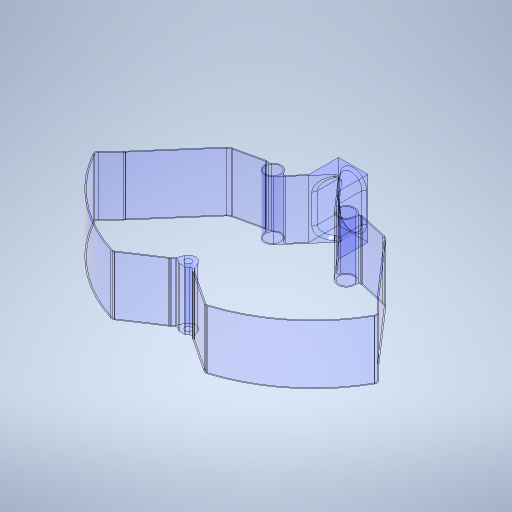
# Autodesk Inventor part: Top Plate
Saved by Autodesk Inventor 2023.2 (Build 272271000, 271)
## iProperties
Created: 2022-12-28
Part Number: Top Plate
Material: UHMW, White
Document SubType Name: Modeling
Designer: Nathan Cai
Mass: 7.48439 g
Surface Area: 194.835 cm^2
Volume: 7.96212 cm^3
Density: 0.94 g/cm^3
Appearance: Clear - Blue
Author: Nathan Cai
Autodesk Inventor part; units mm, degrees
ref_plane "YZ Plane" through (0, 0, 0) normal (1, 0, 0) x (0, 1, 0)
ref_plane "XZ Plane" through (0, 0, 0) normal (0, 1, 0) x (-1, 0, 0)
ref_plane "XY Plane" through (0, 0, 0) normal (0, 0, 1) x (1, 0, 0)
sketch "Sketch1" plane through (0, 0, 0) normal (0, 1, 0) x (-1, 0, 0)
  circle A0 centre (0, 0) radius 73.025
  line L0 (0, 0) -> (0, -73.025) construction
  line L1 (0, 0) -> (-12.6807, -71.9156)
  line L2 (0, 0) -> (12.6807, -71.9156)
  line L3 (0, 0) -> (52.5298, -50.7274)
  line L4 (0, 0) -> (32.0121, -65.6344)
  line L5 (0, 0) -> (72.3143, -10.1631)
  line L6 (0, 0) -> (64.4772, -34.2832)
  line L7 (0, 0) -> (64.4772, 34.2832)
  line L8 (0, 0) -> (72.3143, 10.1631)
  line L9 (0, 0) -> (32.0121, 65.6344)
  line L10 (0, 0) -> (52.5298, 50.7274)
  circle A1 centre (0, 0) radius 69.85
  line L11 (0, 0) -> (-12.6807, 71.9156)
  line L12 (0, 0) -> (12.6807, 71.9156)
  line L13 (0, 0) -> (-52.5298, 50.7274)
  line L14 (0, 0) -> (-32.0121, 65.6344)
  line L15 (0, 0) -> (-72.3143, 10.1631)
  line L16 (0, 0) -> (-64.4772, 34.2832)
  line L17 (0, 0) -> (-64.4772, -34.2832)
  line L18 (0, 0) -> (-72.3143, -10.1631)
  line L19 (0, 0) -> (-32.0121, -65.6344)
  line L20 (0, 0) -> (-52.5298, -50.7274)
  point P0 (30.6202, -62.7808)
  point P1 (50.2459, -48.5219)
  point P2 (52.5298, -50.7274)
  point P3 (64.4772, -34.2832)
  point P4 (61.6739, -32.7926)
  point P5 (69.1702, -9.7212)
  point P6 (72.3143, -10.1631)
  point P7 (72.3143, 10.1631)
  point P8 (69.1702, 9.7212)
  point P9 (61.6739, 32.7926)
  point P10 (52.5298, 50.7274)
  point P11 (50.2459, 48.5219)
  point P12 (30.6202, 62.7808)
  point P13 (-12.1293, -68.7888)
  point P14 (12.1293, -68.7888)
  point P15 (12.6807, -71.9156)
  point P16 (32.0121, -65.6344)
  point P17 (12.1293, 68.7888)
  point P18 (-12.1293, 68.7888)
  point P19 (-12.6807, 71.9156)
  point P20 (-64.4772, 34.2832)
  point P21 (-61.6739, 32.7926)
  point P22 (-69.1702, 9.7212)
  point P23 (-52.5298, -50.7274)
  point P24 (-50.2459, -48.5219)
  point P25 (-30.6202, -62.7808)
  dimension "d0" = 146.05
  dimension "d1" = 10
  dimension "d4" = 360
  dimension "d160" = 139.7
  constraints: 42 end point, 4 coincident, 2 centre point, 2 point on circle, 1 symmetric about line, 1 vertical, 49 other
  measures "d0" diameter of A0
  measures "d1" angle of L0 L1
  measures "d160" diameter of A1
extrude "Extrusion1" add sketch "Sketch1" along normal blind 3.175 contours A0 L5 A1 L8 | A0 L6 A1 L5 | L7 A1 L10 A0 | A1 L5 L8 | L8 L7 A1 | A0 L3 A1 L6 | A1 L6 L5 | L10 A1 L9 A0 | L7 L10 A1 | L2 A1 L1 | L4 A1 L2 | L6 A1 L3 | L3 A1 L4 | L12 A1 L9 | L9 A1 L10 | L14 A1 L11 | L11 A1 L12 | L16 A1 L13 | L13 A1 L14 | L18 A1 L15 | L15 A1 L16 | L20 A1 L17 | L17 A1 L18 | L1 A1 L19 | L19 A1 L20 | L9 A1 L12 A0 | A1 L2 A0 L1 | L1 A0 L19 A1 | A1 L4 A0 L2 | A1 L14 A0 L11 | L13 A0 L14 A1 | A1 L16 A0 L13 | A1 L18 A0 L15 | L17 A0 L18 A1 | A1 L20 A0 L17
sketch "Sketch4" plane through (0, 3.175, 0) normal (0, 1, 0) x (1, 0, 0)
  line L0 (0, 0) -> (0, 66.675) construction
  line L1 (-44.45, 30.1625) -> (44.45, 30.1625) construction
  line L2 (44.45, 30.1625) -> (44.45, 1.5875)
  line L3 (44.45, 1.5875) -> (-44.45, 1.5875) construction
  line L4 (-44.45, 1.5875) -> (-44.45, 30.1625)
  line L5 (-44.45, 30.1625) -> (44.45, 1.5875) construction
  line L6 (44.45, 30.1625) -> (-44.45, 1.5875) construction
  line L7 (-44.45, 15.875) -> (44.45, 15.875) construction
  line L8 (-60.325, 38.1) -> (-44.45, 38.1)
  line L9 (-44.45, 38.1) -> (-44.45, -6.35)
  line L10 (-44.45, -6.35) -> (-60.325, -6.35)
  line L11 (-60.325, -6.35) -> (-60.325, 38.1)
  line L12 (-60.325, 38.1) -> (-44.45, -6.35) construction
  line L13 (-44.45, 38.1) -> (-60.325, -6.35) construction
  line L14 (44.45, 1.5875) -> (44.45, 30.1625)
  line L15 (60.325, 38.1) -> (44.45, 38.1)
  line L16 (44.45, 38.1) -> (44.45, -6.35)
  line L17 (44.45, -6.35) -> (60.325, -6.35)
  line L18 (60.325, -6.35) -> (60.325, 38.1)
  line L19 (60.325, 38.1) -> (44.45, -6.35) construction
  line L20 (44.45, 38.1) -> (60.325, -6.35) construction
  line L21 (38.1, 15.875) -> (38.1, 31.75) construction
  circle A0 centre (38.1, 31.75) radius 1.7526
  circle A1 centre (38.1, 0) radius 1.7526
  circle A2 centre (-38.1, 31.75) radius 1.7526
  circle A3 centre (-38.1, 0) radius 1.7526
  line L22 (-60.325, 38.1) -> (-53.975, 38.1)
  line L23 (-53.975, 38.1) -> (-53.975, 31.75)
  line L24 (-53.975, 31.75) -> (-60.325, 31.75) construction
  line L25 (-60.325, 31.75) -> (-60.325, 38.1)
  line L26 (-53.975, 31.75) -> (-60.325, 28.0838)
  line L27 (-53.975, -6.35) -> (-53.975, 0)
  line L28 (-53.975, 0) -> (-60.325, 3.6662)
  line L29 (53.975, 38.1) -> (53.975, 31.75)
  line L30 (53.975, 31.75) -> (60.325, 28.0838)
  line L31 (53.975, -6.35) -> (53.975, 0)
  line L32 (53.975, 0) -> (60.325, 3.6662)
  line L33 (-38.1, 0) -> (38.1, 0) construction
  circle A4 centre (-15.875, -1.5875) radius 1.7526
  circle A5 centre (15.875, -1.5875) radius 1.7526
  line L34 (-21.3, 28.575) -> (-7.0125, 28.575)
  line L35 (-7.0125, 28.575) -> (-7.0125, 3.175)
  line L36 (-7.0125, 3.175) -> (-21.3, 3.175)
  line L37 (-21.3, 3.175) -> (-21.3, 28.575)
  line L38 (-21.3, 28.575) -> (-7.0125, 3.175) construction
  line L39 (-7.0125, 28.575) -> (-21.3, 3.175) construction
  line L40 (21.3, 28.575) -> (7.0125, 28.575)
  line L41 (7.0125, 28.575) -> (7.0125, 3.175)
  line L42 (7.0125, 3.175) -> (21.3, 3.175)
  line L43 (21.3, 3.175) -> (21.3, 28.575)
  line L44 (21.3, 28.575) -> (7.0125, 3.175) construction
  line L45 (7.0125, 28.575) -> (21.3, 3.175) construction
  circle A6 centre (25.4944, -54.673) radius 3.175
  line L46 (25.4944, -54.673) -> (31.5337, -52.7108) construction
  circle A7 centre (31.5337, -52.7108) radius 1.5875
  line L47 (25.4944, -54.673) -> (25.4944, -51.498) construction
  circle A8 centre (30.2134, -58.922) radius 1.5875
  circle A9 centre (24.1742, -60.8843) radius 1.5875
  circle A10 centre (19.4552, -56.6353) radius 1.5875
  circle A11 centre (20.7755, -50.424) radius 1.5875
  circle A12 centre (26.8147, -48.4618) radius 1.5875
  circle A13 centre (-25.4944, -54.673) radius 3.175
  line L48 (-25.4944, -54.673) -> (-31.5337, -52.7108) construction
  circle A14 centre (-31.5337, -52.7108) radius 1.5875
  line L49 (-25.4944, -54.673) -> (-25.4944, -51.498) construction
  circle A15 centre (-30.2134, -58.922) radius 1.5875
  circle A16 centre (-24.1742, -60.8843) radius 1.5875
  circle A17 centre (-19.4552, -56.6353) radius 1.5875
  circle A18 centre (-20.7755, -50.424) radius 1.5875
  circle A19 centre (-26.8147, -48.4618) radius 1.5875
  circle A20 centre (0, 0) radius 60.325 construction
  line L50 (0, 0) -> (25.4944, -54.673) construction
  circle A21 centre (25.4944, -54.673) radius 9.525 construction
  circle A22 centre (31.75, 38.1) radius 3.175
  circle A23 centre (-31.75, 38.1) radius 3.175
  point P0 (0, 15.875)
  point P1 (-52.3875, 15.875)
  point P2 (52.3875, 15.875)
  point P3 (0, 15.875)
  point P4 (-60.325, 3.6662)
  point P5 (-53.975, -6.35)
  point P6 (-53.975, 38.1)
  point P7 (53.975, -6.35)
  point P8 (60.325, 3.6662)
  point P9 (53.975, 38.1)
  point P10 (-14.1563, 15.875)
  point P11 (14.1563, 15.875)
  dimension "d108" = 6.35
  dimension "d173" = 120.65
  dimension "d30" = 88.9
  dimension "d31" = 28.575
  dimension "d34" = 15.875
  dimension "d35" = 44.45
  dimension "d52" = 6.35
  dimension "d53" = 15.875
  dimension "d54" = 3.5052
  dimension "d63" = 15.875
  dimension "d64" = 6.35
  dimension "d65" = 6.35
  dimension "d66" = 30
  dimension "d78" = 3.5052
  dimension "d79" = 15.875
  dimension "d80" = 17.4625
  dimension "d104" = 14.2875
  dimension "d105" = 25.4
  dimension "d107" = 23.15
  dimension "d111" = 6.35
  dimension "d112" = 3.175
  dimension "d113" = 72
  dimension "d116" = 360
  dimension "d174" = 25
  dimension "d175" = 19.05
  dimension "d176" = 6.35
  dimension "d177" = 22.225
  dimension "d178" = 31.75
  constraints: 102 end point, 33 symmetric about line, 21 centre point, 11 midpoint, 8 parallel, 5 coincident, 5 horizontal, 5 point on line, 4 perpendicular, 4 vertical, 2 vertical alignment, 31 other
  measures "d30" distance of L2.end L3.end
  measures "d31" distance between parallel lines of L3 L1
  measures "d34" distance of L9.end L10.end
  measures "d35" distance of L8.end L9.end
  measures "d52" distance between parallel lines of L16 L21
  measures "d53" distance from line of L7 L21.end
  measures "d54" diameter of A0
  measures "d63" distance of point (0, 15.875) L0.start
  measures "d64" distance of L23.end L24.end
  measures "d65" distance of L22.end L23.end
  measures "d66" angle of L24 L26
  measures "d78" diameter of A4
  measures "d79" distance from line of L0 A4.centre
  measures "d80" distance from line of L7 A4.centre
  measures "d104" distance of L35.end L36.end
  measures "d105" distance of L34.end L35.end
  measures "d107" distance between parallel lines of L4 L37
  measures "d111" distance of L46.start L46.end
  measures "d112" diameter of A7
  measures "d113" angle of L47 L46
  measures "d174" angle of L0 L50
  measures "d175" diameter of A21
  measures "d176" diameter of A22
  measures "d177" vertical distance of point (0, 15.875) A22.centre
  measures "d178" distance from line of L0 A22.centre
extrude "Extrusion2" cut sketch "Sketch4" against normal through all
fillet "Fillet2" radius 4.7625 16 edges at (-44.45, 1.5875, -38.1) (-44.45, 1.5875, 6.35) (44.45, 1.5875, 6.35) (44.45, 1.5875, -38.1) (-21.3, 1.5875, -28.575) (-7.0125, 1.5875, -28.575) (-7.0125, 1.5875, -3.175) (-21.3, 1.5875, -3.175) (7.0125, 1.5875, -28.575) (21.3, 1.5875, -28.575) (21.3, 1.5875, -3.175) (7.0125, 1.5875, -3.175) (60.325, 1.5875, -38.1) (60.325, 1.5875, 6.35) (-60.325, 1.5875, -38.1) (-60.325, 1.5875, 6.35)
sketch "Sketch5" plane through (0, 3.175, 0) normal (0, 1, 0) x (1, 0, 0)
  line L0 (0, 0) -> (0, 66.675) construction
  circle A0 centre (0, 50.8) radius 22.225
  arc A1 (32.0121, 65.6344) -> (-32.0121, 65.6344) centre (0, 0) ccw projected
  circle A2 centre (0, 50.8) radius 17.4625 construction
  circle A3 centre (-24.6063, 60.325) radius 1.7526
  circle A4 centre (-24.6063, 60.325) radius 3.175 construction
  circle A5 centre (-22.225, 34.925) radius 3.175 construction
  circle A6 centre (-22.225, 34.925) radius 1.7526
  circle A7 centre (24.6063, 60.325) radius 1.7526
  circle A8 centre (24.6063, 60.325) radius 3.175 construction
  circle A9 centre (22.225, 34.925) radius 3.175 construction
  circle A10 centre (22.225, 34.925) radius 1.7526
  arc A11 (32.0121, 65.6344) -> (-32.0121, 65.6344) centre (0, 0) ccw projected
  line L1 (-19.05, 70.4964) -> (-21.8767, 54.7195)
  line L2 (19.05, 70.4964) -> (21.8767, 54.7195)
  circle A12 centre (0, 28.575) radius 4.7625
  line L3 (0, 33.3375) -> (0, 23.8125) construction
  line L4 (-4.7625, 33.3375) -> (-4.7625, 23.8125)
  line L5 (4.7625, 23.8125) -> (4.7625, 33.3375)
  arc A13 (4.7625, 33.3375) -> (-4.7625, 33.3375) centre (0, 33.3375) ccw
  arc A14 (-4.7625, 23.8125) -> (4.7625, 23.8125) centre (0, 23.8125) ccw
  point P0 (-30.5456, -66.3296)
  point P1 (12.6807, -71.9156)
  point P2 (64.4772, -34.2832)
  point P3 (-72.5223, -8.5536)
  point P4 (-19.05, 70.4964)
  point P5 (0, 73.025)
  point P6 (21.8767, 54.7195)
  point P7 (19.05, 70.4964)
  point P8 (-4.7351, 29.0853)
  point P9 (4.7351, 29.0853)
  point P10 (0, 19.05)
  point P11 (4.7625, 28.575)
  point P12 (-4.7625, 28.575)
  dimension "d39" = 34.925
  dimension "d40" = 44.45
  dimension "d41" = 3.5052
  dimension "d42" = 6.35
  dimension "d43" = 9.525
  dimension "d44" = 24.6062
  dimension "d45" = 6.35
  dimension "d46" = 3.5052
  dimension "d47" = 15.875
  dimension "d48" = 22.225
  dimension "d74" = 19.05
  dimension "d102" = 9.525
  dimension "d103" = 9.525
  constraints: 14 end point, 13 centre point, 8 point on circle, 7 tangent, 6 symmetric about line, 5 coincident, 3 point on line, 1 midpoint, 1 parallel, 1 vertical, 4 other
  measures "d39" diameter of A2
  measures "d40" diameter of A0
  measures "d41" diameter of A3
  measures "d42" diameter of A4
  measures "d43" vertical distance of A0.centre A3.centre
  measures "d44" horizontal distance of A0.centre A3.centre
  measures "d45" diameter of A5
  measures "d46" diameter of A6
  measures "d47" vertical distance of A0.centre A6.centre
  measures "d48" horizontal distance of A0.centre A6.centre
  measures "d74" distance from line of L0 L1.start
  measures "d102" diameter of A12
  measures "d103" distance of point (0, 19.05) A12.centre
extrude "Extrusion3" cut sketch "Sketch5" against normal blind 25.4 contours A0 L5 A13 L4 | A0 A1 L2 | A0 A12 L4 A13 L5 | A0 L1 A1 | A12 A0 | A0 A12 | L5 A14 L4 A12 | A3 | A6 | A7 | A10
sketch "Sketch6" plane through (0, 0, 0) normal (0, -1, 0) x (1, 0, 0)
  point P0 (11.8537, 67.2254)
  point P1 (-11.8537, 67.2254)
hole "Hole3" at (11.8537, 0, 67.2254) at (-11.8537, 0, 67.2254) direction (0, 1, 0) diameter 3.5052 end through all
sketch "Sketch7" plane through (0, 3.175, 0) normal (0, 1, 0) x (1, 0, 0)
  arc A0 (12.158, -68.9514) -> (11.3889, -68.9153) centre (11.8537, -67.2254) ccw projected
  circle A1 centre (11.8537, -67.2254) radius 3.302
  arc A2 (-11.3889, -68.9153) -> (-12.158, -68.9514) centre (-11.8537, -67.2254) ccw projected
  circle A3 centre (-11.8537, -67.2254) radius 3.302
  circle A4 centre (11.8537, -67.2254) radius 1.7526
  circle A5 centre (-11.8537, -67.2254) radius 1.7526
  point P0 (0, 0)
  point P1 (12.158, -68.9514)
  point P2 (11.3889, -68.9153)
  dimension "d67" = 6.604
  dimension "d68" = 6.604
  constraints: 4 coincident, 3 centre point, 1 concentric, 3 other
  measures "d67" diameter of A1
  measures "d68" diameter of A3
extrude "Extrusion4" add sketch "Sketch7" against normal up to surface (3.175 mm away)
fillet "Fillet4" radius 1.5875 24 edges at (-12.6807, 1.5875, 71.9156) (-12.427, 1.5875, 70.4773) (-9.235, 1.5875, 69.2368) (12.6807, 1.5875, 71.9156) (12.427, 1.5875, 70.4773) (9.235, 1.5875, 69.2368) (69.1702, 1.5875, 9.7212) (72.3143, 1.5875, 10.1631) (64.4772, 1.5875, 34.2832) (61.6739, 1.5875, 32.7926) (30.6202, 1.5875, -62.7808) (32.0121, 1.5875, -65.6344) (52.5298, 1.5875, -50.7274) (50.2459, 1.5875, -48.5219) (-32.0121, 1.5875, -65.6344) (-30.6202, 1.5875, -62.7808) (-52.5298, 1.5875, -50.7274) (-50.2459, 1.5875, -48.5219) (-72.3143, 1.5875, 10.1631) (-69.1702, 1.5875, 9.7212) (-61.6739, 1.5875, 32.7926) (-64.4772, 1.5875, 34.2832) (-4.7351, 1.5875, -29.0853) (4.7351, 1.5875, -29.0853)
fillet "Fillet5" radius 3.175 2 edges at (19.05, 1.5875, -70.4964) (-19.05, 1.5875, -70.4964)
thicken "Thicken1" operation cut thickness 0.25 both sides no extend neighbours no toward (-0.8477101, 0, -0.5304598) faces at (61.904, 2.1167, 38.7368) (63.0601, 1.0583, 33.5296) (63.8199, 1.0583, 34.4266) (13.1942, 1.0583, 71.6582) (62.9587, 1.0583, 33.4709) (12.2225, 1.0583, 70.9396) (66.7871, 2.1167, 20.4576) (9.8443, 2.1167, 69.8457) (70.7248, 1.0583, 9.9397) (69.8129, 1.0583, 10.0825) (8.7126, 2.1167, 69.3268) (70.965, 1.0583, 9.9551) (6.579, 2.1167, 69.5395) (62.1056, 2.1167, -38.4128) (-8.7126, 2.1167, 69.3268) (51.3752, 1.0583, -49.6125) (52.5834, 1.0583, -50.0545) (-9.8443, 1.0583, 69.8457) (50.9955, 1.0583, -49.3411) (-11.7264, 1.0583, 70.5997) (40.0946, 2.1167, -57.1965) (-12.915, 1.0583, 71.5521) (31.3084, 1.0583, -64.1918) (31.1624, 1.0583, -63.2804) (-45.5793, 2.1167, 57.0541) (31.3571, 1.0583, -64.302) (-63.06, 1.0583, 33.5296) (-63.6672, 1.0583, 34.1) (24.8679, 2.1167, -68.6603) (-62.2411, 1.0583, 31.857) (-63.4147, 2.1167, 29.2848) (-70.7249, 1.0583, 9.9397) (-70.2583, 1.0583, 9.9434) (-72.3414, 1.0583, 9.1242) (-72.823, 2.1167, -5.4282) (-51.3752, 1.0583, -49.6124) (-51.8764, 1.0583, -49.9396) (-49.8575, 1.0583, -49.222) (-42.0072, 2.1167, -55.807) (-31.3084, 1.0583, -64.1918) (-31.8083, 1.0583, -62.207) (-31.1844, 1.0583, -65.7948) (-29.847, 2.1167, -66.6469) (19.9211, 2.1167, -65.8489) (21.2411, 2.1167, -58.2668) (13.984, 1.0583, -33.5258) (5.2423, 1.0583, -28.987) (4.7625, 2.1167, -25.1583) (-4.3814, 1.0583, -21.9458) (-4.7625, 1.0583, -26.5041) (-5.421, 1.0583, -29.1371) (-19.7168, 1.0583, -40.5434) (-20.6056, 2.1167, -61.8142) (-19.9361, 2.1167, -65.6043)
sketch "Sketch11" plane through (0, 3.175, 0) normal (0, 1, 0) x (1, 0, 0)
  line L0 (-26.9875, -14.2875) -> (-7.9375, -14.2875) construction
  line L1 (-26.9875, -16.6688) -> (-7.9375, -16.6688)
  line L2 (-7.9375, -11.9062) -> (-26.9875, -11.9063)
  arc A0 (-26.9875, -11.9063) -> (-26.9875, -16.6688) centre (-26.9875, -14.2875) ccw
  arc A1 (-7.9375, -16.6688) -> (-7.9375, -11.9062) centre (-7.9375, -14.2875) ccw
  line L3 (-17.4625, -14.2875) -> (-17.4625, -39.6875) construction
  line L4 (-23.8125, -26.9875) -> (-11.1125, -26.9875) construction
  line L5 (-23.8125, -29.3688) -> (-11.1125, -29.3687)
  line L6 (-11.1125, -24.6062) -> (-23.8125, -24.6062)
  arc A2 (-23.8125, -24.6062) -> (-23.8125, -29.3688) centre (-23.8125, -26.9875) ccw
  arc A3 (-11.1125, -29.3687) -> (-11.1125, -24.6062) centre (-11.1125, -26.9875) ccw
  line L7 (-30.1625, -39.6875) -> (-4.7625, -39.6875) construction
  line L8 (-30.1625, -42.0688) -> (-4.7625, -42.0688)
  line L9 (-4.7625, -37.3062) -> (-30.1625, -37.3063)
  arc A4 (-30.1625, -37.3063) -> (-30.1625, -42.0688) centre (-30.1625, -39.6875) ccw
  arc A5 (-4.7625, -42.0688) -> (-4.7625, -37.3062) centre (-4.7625, -39.6875) ccw
  circle A6 centre (-11.1125, -33.3375) radius 2.3813
  line L10 (-17.4625, -39.6875) -> (-17.4625, -14.2875) construction
  line L11 (-15.0813, -39.6875) -> (-15.0812, -14.2875)
  line L12 (-19.8438, -14.2875) -> (-19.8438, -39.6875)
  arc A7 (-19.8438, -39.6875) -> (-15.0813, -39.6875) centre (-17.4625, -39.6875) ccw construction
  arc A8 (-15.0812, -14.2875) -> (-19.8438, -14.2875) centre (-17.4625, -14.2875) ccw construction
  line L13 (20.6375, -14.2875) -> (20.6375, -39.6875) construction
  circle A9 centre (14.2875, -14.2875) radius 2.3813 construction
  line L14 (15.875, -20.6375) -> (15.875, -26.9875) construction
  line L15 (13.4938, -20.6375) -> (13.4938, -26.9875)
  line L16 (18.2563, -26.9875) -> (18.2563, -20.6375)
  arc A10 (18.2563, -20.6375) -> (13.4938, -20.6375) centre (15.875, -20.6375) ccw
  arc A11 (13.4938, -26.9875) -> (18.2563, -26.9875) centre (15.875, -26.9875) ccw
  line L17 (15.875, -20.6375) -> (25.4, -20.6375) construction
  line L18 (15.875, -23.0187) -> (25.4, -23.0187)
  line L19 (25.4, -18.2562) -> (15.875, -18.2562)
  arc A12 (15.875, -18.2562) -> (15.875, -23.0187) centre (15.875, -20.6375) ccw
  arc A13 (25.4, -23.0187) -> (25.4, -18.2562) centre (25.4, -20.6375) ccw
  line L20 (15.875, -26.9875) -> (25.4, -26.9875) construction
  line L21 (15.875, -24.6062) -> (25.4, -24.6062)
  line L22 (25.4, -29.3687) -> (15.875, -29.3687)
  arc A14 (15.875, -24.6062) -> (15.875, -29.3687) centre (15.875, -26.9875) ccw
  arc A15 (25.4, -29.3687) -> (25.4, -24.6062) centre (25.4, -26.9875) ccw
  circle A16 centre (26.9875, -14.2875) radius 2.3813 construction
  line L23 (26.9875, -14.2875) -> (30.1625, -8.7882) construction
  line L24 (29.0497, -15.4781) -> (32.2247, -9.9789)
  line L25 (28.1003, -7.5976) -> (24.9253, -13.0969)
  arc A17 (24.9253, -13.0969) -> (29.0497, -15.4781) centre (26.9875, -14.2875) ccw
  arc A18 (32.2247, -9.9789) -> (28.1003, -7.5976) centre (30.1625, -8.7882) ccw
  line L26 (26.9875, -14.2875) -> (33.3375, -14.2875) construction
  line L27 (14.2875, -14.2875) -> (11.1125, -8.7882) construction
  line L28 (16.3497, -13.0969) -> (13.1747, -7.5976)
  line L29 (9.0503, -9.9789) -> (12.2253, -15.4781)
  arc A19 (12.2253, -15.4781) -> (16.3497, -13.0969) centre (14.2875, -14.2875) ccw
  arc A20 (13.1747, -7.5976) -> (9.0503, -9.9789) centre (11.1125, -8.7882) ccw
  line L30 (14.2875, -14.2875) -> (20.6375, -14.2875) construction
  line L31 (11.1125, -33.3375) -> (11.1125, -39.6875) construction
  line L32 (8.7313, -33.3375) -> (8.7313, -39.6875)
  line L33 (13.4938, -39.6875) -> (13.4938, -33.3375)
  arc A21 (13.4938, -33.3375) -> (8.7313, -33.3375) centre (11.1125, -33.3375) ccw
  arc A22 (8.7313, -39.6875) -> (13.4938, -39.6875) centre (11.1125, -39.6875) ccw
  line L34 (17.4625, -33.3375) -> (17.4625, -39.6875) construction
  line L35 (15.0813, -33.3375) -> (15.0813, -39.6875)
  line L36 (19.8438, -39.6875) -> (19.8438, -33.3375)
  arc A23 (19.8438, -33.3375) -> (15.0813, -33.3375) centre (17.4625, -33.3375) ccw
  arc A24 (15.0813, -39.6875) -> (19.8438, -39.6875) centre (17.4625, -39.6875) ccw
  line L37 (17.4625, -39.6875) -> (30.1625, -39.6875) construction
  line L38 (17.4625, -37.3062) -> (30.1625, -37.3062)
  line L39 (30.1625, -42.0688) -> (17.4625, -42.0688)
  arc A25 (17.4625, -37.3062) -> (17.4625, -42.0688) centre (17.4625, -39.6875) ccw
  arc A26 (30.1625, -42.0688) -> (30.1625, -37.3062) centre (30.1625, -39.6875) ccw
  circle A27 centre (23.8125, -33.3375) radius 2.3813
  circle A28 centre (30.1625, -33.3375) radius 2.3813
  line L40 (17.4625, -33.3375) -> (30.1625, -33.3375) construction
  line L41 (30.1625, -33.3375) -> (30.1625, -39.6875) construction
  arc A29 (53.6121, -36.9069) -> (36.9069, -53.6121) centre (52.759, -52.759) ccw construction
  arc A30 (53.7828, -33.7365) -> (33.7365, -53.7828) centre (52.759, -52.759) ccw
  arc A31 (53.4415, -40.0774) -> (40.0774, -53.4415) centre (52.759, -52.759) ccw
  arc A32 (53.4415, -40.0774) -> (53.7828, -33.7365) centre (53.6121, -36.9069) ccw
  arc A33 (33.7365, -53.7828) -> (40.0774, -53.4415) centre (36.9069, -53.6121) ccw
  circle A34 centre (0, 0) radius 65.0875 construction
  line L42 (0, 0) -> (41.5337, -41.5337) construction
  circle A35 centre (0, -64.525) radius 3 projected
  line L43 (0, 0) -> (0, -64.525) construction
  circle A36 centre (52.759, -52.759) radius 9.525
  arc A37 (-36.9069, -53.6121) -> (-53.6121, -36.9069) centre (-52.759, -52.759) ccw construction
  arc A38 (-33.7365, -53.7828) -> (-53.7828, -33.7365) centre (-52.759, -52.759) ccw
  arc A39 (-40.0774, -53.4415) -> (-53.4415, -40.0774) centre (-52.759, -52.759) ccw
  arc A40 (-53.7828, -33.7365) -> (-53.4415, -40.0774) centre (-53.6121, -36.9069) ccw
  arc A41 (-40.0774, -53.4415) -> (-33.7365, -53.7828) centre (-36.9069, -53.6121) ccw
  circle A42 centre (-52.759, -52.759) radius 9.525
  point P0 (-17.4625, -26.9875)
  point P1 (15.875, -23.8125)
  point P2 (20.6375, -20.6375)
  point P3 (20.6375, -26.9875)
  point P4 (20.6375, -26.9875)
  point P5 (28.575, -11.5379)
  point P6 (12.7, -11.5379)
  point P7 (11.1125, -36.5125)
  point P8 (17.4625, -36.5125)
  point P9 (23.8125, -39.6875)
  point P10 (-19.8438, -29.3688)
  point P11 (-19.8438, -37.3062)
  point P12 (-15.0813, -37.3062)
  point P13 (-15.0813, -29.3687)
  point P14 (-15.0812, -24.6062)
  point P15 (-15.0812, -16.6688)
  point P16 (-19.8438, -16.6688)
  point P17 (-19.8438, -24.6062)
  point P18 (15.875, -18.2562)
  point P19 (18.2563, -24.6062)
  point P20 (18.2563, -23.0187)
  point P21 (19.8438, -37.3062)
  dimension "d118" = 9.525
  dimension "d119" = 4.7625
  dimension "d120" = 25.4
  dimension "d121" = 2.3813
  dimension "d122" = 6.35
  dimension "d123" = 2.3813
  dimension "d124" = 12.7
  dimension "d125" = 4.7625
  dimension "d126" = 6.35
  dimension "d127" = 6.35
  dimension "d128" = 26.9875
  dimension "d129" = 17.4625
  dimension "d130" = 2.3813
  dimension "d131" = 20.6375
  dimension "d132" = 4.7625
  dimension "d133" = 3.175
  dimension "d134" = 4.7625
  dimension "d135" = 4.7625
  dimension "d136" = 2.3813
  dimension "d137" = 26.9875
  dimension "d138" = 6.35
  dimension "d139" = 6.35
  dimension "d140" = 6.35
  dimension "d141" = 60
  dimension "d142" = 6.35
  dimension "d143" = 120
  dimension "d144" = 2.3813
  dimension "d145" = 2.3813
  dimension "d146" = 3.175
  dimension "d147" = 25.4
  dimension "d148" = 6.35
  dimension "d149" = 6.35
  dimension "d150" = 4.7625
  dimension "d151" = 4.7625
  dimension "d152" = 6.35
  dimension "d155" = 6.35
  dimension "d156" = 130.175
  dimension "d157" = 15.875
  dimension "d158" = 45
  dimension "d159" = 19.05
  constraints: 112 end point, 74 point on circle, 53 tangent, 42 centre point, 17 equal length, 16 midpoint, 8 symmetric about line, 6 horizontal, 6 point on line, 5 vertical, 4 coincident, 3 perpendicular, 2 concentric, 6 other
  measures "d118" distance of L3.start L0.end
  measures "d119" diameter of A1
  measures "d120" distance of L3.start L3.end
  measures "d121" radius of A3
  measures "d122" distance of L4.end point (-17.463, -26.988)
  measures "d123" radius of A5
  measures "d124" distance of L7.end L3.end
  measures "d125" diameter of A6
  measures "d126" distance from line of L3 A6.centre
  measures "d127" distance from line of L4 A6.centre
  measures "d128" vertical distance of point (0, 0) point (-17.463, -26.988)
  measures "d129" horizontal distance of point (0, 0) point (-17.463, -26.988)
  measures "d130" radius of A8
  measures "d131" horizontal distance of point (20.638, -26.988) point (0, 0)
  measures "d132" diameter of A9
  measures "d133" distance of point (15.875, -23.812) L14.end
  measures "d134" diameter of A16
  measures "d135" distance between parallel lines of L13 L14
  measures "d136" radius of A13
  measures "d137" vertical distance of point (0, 0) point (20.638, -26.988)
  measures "d138" distance from line of L13 L27.start
  measures "d139" distance from line of L13 L23.start
  measures "d140" distance of L23.start L23.end
  measures "d141" angle of L26 L23
  measures "d142" distance of L27.start L27.end
  measures "d143" angle of L30 L27
  measures "d144" radius of A26
  measures "d145" radius of A21
  measures "d146" distance between parallel lines of L34 L13
  measures "d147" distance of L13.start L13.end
  measures "d148" distance of L34.end L34.start
  measures "d149" distance of L37.end point (23.813, -39.688)
  measures "d150" diameter of A27
  measures "d151" diameter of A28
  measures "d152" distance between parallel lines of L34 L31
  measures "d155" diameter of A33
  measures "d156" diameter of A34
  measures "d157" radius of A29
  measures "d158" angle of L43 L42
  measures "d159" diameter of A36
extrude "Extrusion5" [suppressed]
sketch "Sketch13" plane through (0, 3.175, 0) normal (0, 1, 0) x (1, 0, 0)
  circle A0 centre (0, -65.0875) radius 7.9375 construction
  line L0 (0, 0) -> (0, -73.025) construction
  circle A1 centre (0, -53.975) radius 3.175
  circle A2 centre (0, -53.975) radius 1.7526
  circle A3 centre (0, 0) radius 73.025 construction
  dimension "d168" = 15.875
  dimension "d212" = 146.05
  dimension "d170" = 6.35
  dimension "d210" = 3.5052
  constraints: 2 centre point, 2 coincident, 2 end point, 2 point on line, 2 vertical alignment, 1 vertical, 4 other
  measures "d170" diameter of A1
  measures "d210" diameter of A2
extrude "Extrusion6" cut sketch "Sketch13" against normal through all contours A2
sketch "Sketch14" plane through (0, 3.175, 0) normal (0, 1, 0) x (1, 0, 0)
  arc A0 (-8.4203, -69.0888) -> (-9.8493, -69.5271) centre (-8.6426, -70.9128) ccw projected
  arc A1 (-8.4203, -69.0888) -> (8.4203, -69.0888) centre (0, 0) ccw projected
  arc A2 (9.8493, -69.5271) -> (8.4203, -69.0888) centre (8.6426, -70.9128) ccw projected
  arc A3 (9.8493, -69.5271) -> (11.3791, -70.2403) centre (11.8537, -67.2254) ccw projected
  arc A4 (12.5534, -70.9399) -> (11.3791, -70.2403) centre (11.0933, -72.0555) ccw projected
  arc A5 (12.5534, -70.9399) -> (13.8711, -71.4408) centre (13.6162, -70.1278) ccw projected
  arc A6 (13.8711, -71.4408) -> (63.4814, -35.5853) centre (0, 0) ccw projected
  arc A7 (63.4814, -35.5853) -> (62.9426, -33.7503) centre (62.3147, -34.9313) ccw projected
  arc A8 (62.1641, -31.3015) -> (62.9426, -33.7503) centre (63.8053, -32.1279) ccw projected
  arc A9 (62.1641, -31.3015) -> (68.6904, -11.2157) centre (0, 0) ccw projected
  arc A10 (70.7596, -9.6922) -> (68.6904, -11.2157) centre (70.5039, -11.5118) ccw projected
  arc A11 (70.7596, -9.6922) -> (72.274, -8.5243) centre (70.9457, -8.3677) ccw projected
  arc A12 (72.274, -8.5243) -> (53.4604, 49.3779) centre (0, 0) ccw projected
  arc A13 (53.4604, 49.3779) -> (51.5488, 49.4326) centre (52.4779, 48.4705) ccw projected
  arc A14 (48.9793, 49.4489) -> (51.5488, 49.4326) centre (50.2724, 50.7544) ccw projected
  arc A15 (48.9793, 49.4489) -> (31.8932, 61.8626) centre (0, 0) ccw projected
  arc A16 (31.0837, 64.3013) -> (31.8932, 61.8626) centre (32.7352, 63.4958) ccw projected
  arc A17 (31.0837, 64.3013) -> (30.441, 66.1025) centre (29.8816, 64.8877) ccw projected
  arc A18 (30.441, 66.1025) -> (24.0624, 68.6819) centre (0, 0) ccw projected
  arc A19 (24.0624, 68.6819) -> (20.2161, 65.4056) centre (23.0952, 65.9214) ccw projected
  line L0 (20.2161, 65.4056) -> (22.1227, 54.7636) projected
  arc A20 (5.9933, 29.1388) -> (22.1227, 54.7636) centre (0, 50.8) ccw projected
  arc A21 (5.9933, 29.1388) -> (5.0125, 27.8498) centre (6.35, 27.8498) ccw projected
  line L1 (5.0125, 27.8498) -> (5.0125, 23.8125) projected
  arc A22 (-5.0125, 23.8125) -> (5.0125, 23.8125) centre (0, 23.8125) ccw projected
  line L2 (-5.0125, 23.8125) -> (-5.0125, 27.8498) projected
  arc A23 (-5.0125, 27.8498) -> (-5.9933, 29.1388) centre (-6.35, 27.8498) ccw projected
  arc A24 (-22.1227, 54.7636) -> (-5.9933, 29.1388) centre (0, 50.8) ccw projected
  line L3 (-22.1227, 54.7636) -> (-20.2161, 65.4056) projected
  arc A25 (-20.2161, 65.4056) -> (-24.0624, 68.6819) centre (-23.0952, 65.9214) ccw projected
  arc A26 (-24.0624, 68.6819) -> (-30.441, 66.1025) centre (0, 0) ccw projected
  arc A27 (-30.441, 66.1025) -> (-31.0837, 64.3013) centre (-29.8816, 64.8877) ccw projected
  arc A28 (-31.8932, 61.8626) -> (-31.0837, 64.3013) centre (-32.7352, 63.4958) ccw projected
  arc A29 (-31.8932, 61.8626) -> (-48.9793, 49.4489) centre (0, 0) ccw projected
  arc A30 (-51.5488, 49.4326) -> (-48.9793, 49.4489) centre (-50.2724, 50.7544) ccw projected
  arc A31 (-51.5488, 49.4326) -> (-53.4604, 49.3779) centre (-52.4779, 48.4705) ccw projected
  arc A32 (-53.4604, 49.3779) -> (-72.274, -8.5243) centre (0, 0) ccw projected
  arc A33 (-72.274, -8.5243) -> (-70.7596, -9.6922) centre (-70.9457, -8.3677) ccw projected
  arc A34 (-68.6904, -11.2157) -> (-70.7596, -9.6922) centre (-70.5039, -11.5118) ccw projected
  arc A35 (-68.6904, -11.2157) -> (-62.1641, -31.3015) centre (0, 0) ccw projected
  arc A36 (-62.9426, -33.7503) -> (-62.1641, -31.3015) centre (-63.8053, -32.1279) ccw projected
  arc A37 (-62.9426, -33.7503) -> (-63.4814, -35.5853) centre (-62.3147, -34.9313) ccw projected
  arc A38 (-63.4814, -35.5853) -> (-13.8711, -71.4408) centre (0, 0) ccw projected
  arc A39 (-13.8711, -71.4408) -> (-12.5534, -70.9399) centre (-13.6162, -70.1278) ccw projected
  arc A40 (-11.3791, -70.2403) -> (-12.5534, -70.9399) centre (-11.0933, -72.0555) ccw projected
  arc A41 (-11.3791, -70.2403) -> (-9.8493, -69.5271) centre (-11.8537, -67.2254) ccw projected
  circle A42 centre (11.8537, -67.2254) radius 1.7526 projected
  circle A43 centre (-11.8537, -67.2254) radius 1.7526 projected
  circle A44 centre (31.75, 38.1) radius 3.175 projected
  circle A45 centre (25.4944, -54.673) radius 3.175 projected
  circle A46 centre (24.1742, -60.8843) radius 1.5875 projected
  circle A47 centre (-31.5337, -52.7108) radius 1.5875 projected
  line L4 (-7.0125, 23.8125) -> (-7.0125, 7.9375) projected
  arc A48 (-11.775, 3.175) -> (-7.0125, 7.9375) centre (-11.775, 7.9375) ccw projected
  line L5 (-11.775, 3.175) -> (-16.5375, 3.175) projected
  arc A49 (-21.3, 7.9375) -> (-16.5375, 3.175) centre (-16.5375, 7.9375) ccw projected
  line L6 (-21.3, 7.9375) -> (-21.3, 23.8125) projected
  arc A50 (-16.5375, 28.575) -> (-21.3, 23.8125) centre (-16.5375, 23.8125) ccw projected
  line L7 (-16.5375, 28.575) -> (-11.775, 28.575) projected
  arc A51 (-7.0125, 23.8125) -> (-11.775, 28.575) centre (-11.775, 23.8125) ccw projected
  line L8 (49.2125, 38.1) -> (55.5625, 38.1) projected
  arc A52 (60.325, 33.3375) -> (55.5625, 38.1) centre (55.5625, 33.3375) ccw projected
  line L9 (60.325, 33.3375) -> (60.325, -1.5875) projected
  arc A53 (55.5625, -6.35) -> (60.325, -1.5875) centre (55.5625, -1.5875) ccw projected
  line L10 (55.5625, -6.35) -> (49.2125, -6.35) projected
  arc A54 (44.45, -1.5875) -> (49.2125, -6.35) centre (49.2125, -1.5875) ccw projected
  line L11 (44.45, -1.5875) -> (44.45, 33.3375) projected
  arc A55 (49.2125, 38.1) -> (44.45, 33.3375) centre (49.2125, 33.3375) ccw projected
  circle A56 centre (38.1, 0) radius 1.7526 projected
  circle A57 centre (-38.1, 0) radius 1.7526 projected
  circle A58 centre (15.875, -1.5875) radius 1.7526 projected
  circle A59 centre (-30.2134, -58.922) radius 1.5875 projected
  circle A60 centre (-24.1742, -60.8843) radius 1.5875 projected
  circle A61 centre (26.8147, -48.4618) radius 1.5875 projected
  circle A62 centre (30.2134, -58.922) radius 1.5875 projected
  circle A63 centre (-31.75, 38.1) radius 3.175 projected
  circle A64 centre (31.5337, -52.7108) radius 1.5875 projected
  circle A65 centre (-25.4944, -54.673) radius 3.175 projected
  circle A66 centre (-19.4552, -56.6353) radius 1.5875 projected
  line L12 (21.3, 23.8125) -> (21.3, 7.9375) projected
  arc A67 (16.5375, 3.175) -> (21.3, 7.9375) centre (16.5375, 7.9375) ccw projected
  line L13 (16.5375, 3.175) -> (11.775, 3.175) projected
  arc A68 (7.0125, 7.9375) -> (11.775, 3.175) centre (11.775, 7.9375) ccw projected
  line L14 (7.0125, 7.9375) -> (7.0125, 23.8125) projected
  arc A69 (11.775, 28.575) -> (7.0125, 23.8125) centre (11.775, 23.8125) ccw projected
  line L15 (11.775, 28.575) -> (16.5375, 28.575) projected
  arc A70 (21.3, 23.8125) -> (16.5375, 28.575) centre (16.5375, 23.8125) ccw projected
  line L16 (-44.45, 33.3375) -> (-44.45, -1.5875) projected
  arc A71 (-49.2125, -6.35) -> (-44.45, -1.5875) centre (-49.2125, -1.5875) ccw projected
  line L17 (-49.2125, -6.35) -> (-55.5625, -6.35) projected
  arc A72 (-60.325, -1.5875) -> (-55.5625, -6.35) centre (-55.5625, -1.5875) ccw projected
  line L18 (-60.325, -1.5875) -> (-60.325, 33.3375) projected
  arc A73 (-55.5625, 38.1) -> (-60.325, 33.3375) centre (-55.5625, 33.3375) ccw projected
  line L19 (-55.5625, 38.1) -> (-49.2125, 38.1) projected
  arc A74 (-44.45, 33.3375) -> (-49.2125, 38.1) centre (-49.2125, 33.3375) ccw projected
  circle A75 centre (38.1, 31.75) radius 1.7526 projected
  circle A76 centre (-38.1, 31.75) radius 1.7526 projected
  circle A77 centre (-15.875, -1.5875) radius 1.7526 projected
  circle A78 centre (-26.8147, -48.4618) radius 1.5875 projected
  circle A79 centre (-20.7755, -50.424) radius 1.5875 projected
  circle A80 centre (19.4552, -56.6353) radius 1.5875 projected
  circle A81 centre (20.7755, -50.424) radius 1.5875 projected
  circle A82 centre (22.225, 34.925) radius 1.7526 projected
  circle A83 centre (-22.225, 34.925) radius 1.7526 projected
  circle A84 centre (24.6063, 60.325) radius 1.7526 projected
  circle A85 centre (-24.6063, 60.325) radius 1.7526 projected
  circle A86 centre (0, 0) radius 73.025
  line L20 (0, 0) -> (0, -73.025) construction
  circle A87 centre (0, -65.0875) radius 7.9375 construction
  circle A88 centre (0, -65.0875) radius 9.525
  circle A89 centre (0, 0) radius 69.85
  circle A90 centre (61.9019, -20.1131) radius 9.525
  circle A91 centre (38.2575, 52.6569) radius 9.525
  circle A92 centre (-38.2575, 52.6569) radius 9.525
  circle A93 centre (-61.9019, -20.1131) radius 9.525
  circle A94 centre (-15.875, -1.5875) radius 3.175
  circle A95 centre (15.875, -1.5875) radius 3.175
  circle A96 centre (-38.1, 0) radius 1.7526 projected
  circle A97 centre (-38.1, 0) radius 4.7625
  line L21 (-55.1667, -26.8483) -> (-61.4776, -33.1592)
  line L22 (-16.5662, 1.5114) -> (-32.8016, -2.1097)
  line L23 (-34.5063, -3.1251) -> (-54.7144, -26.3634)
  arc A98 (-32.8016, -2.1097) -> (-34.5063, -3.1251) centre (-32.1104, -5.2086) ccw
  line L24 (-18.4431, 0.2795) -> (-32.6288, -2.8844)
  arc A99 (-32.6288, -2.8844) -> (-33.9073, -3.646) centre (-32.1104, -5.2086) ccw
  line L25 (-33.9073, -3.646) -> (-60.7364, -34.498)
  line L26 (-5.425, 7.9375) -> (-5.425, 23.8125)
  arc A100 (-5.425, 23.8125) -> (-11.775, 30.1625) centre (-11.775, 23.8125) ccw
  line L27 (-11.775, 30.1625) -> (-16.5375, 30.1625)
  arc A101 (-16.5375, 30.1625) -> (-22.8875, 23.8125) centre (-16.5375, 23.8125) ccw
  line L28 (-22.8875, 23.8125) -> (-22.8875, 7.9375)
  arc A102 (-22.8875, 7.9375) -> (-16.5375, 1.5875) centre (-16.5375, 7.9375) ccw
  line L29 (-16.5375, 1.5875) -> (-11.775, 1.5875)
  arc A103 (-11.775, 1.5875) -> (-5.425, 7.9375) centre (-11.775, 7.9375) ccw
  line L30 (-7.0125, 23.8125) -> (-7.0125, 7.9375) projected
  line L31 (-13.4831, -3.6754) -> (0, 11.7707)
  line L32 (0, 0) -> (0, 69.85) construction
  line L33 (55.1667, -26.8483) -> (61.4776, -33.1592)
  line L34 (16.5662, 1.5114) -> (32.8016, -2.1097)
  line L35 (34.5063, -3.1251) -> (54.7144, -26.3634)
  arc A104 (34.5063, -3.1251) -> (32.8016, -2.1097) centre (32.1104, -5.2086) ccw
  line L36 (18.4431, 0.2795) -> (32.6288, -2.8844)
  arc A105 (33.9073, -3.646) -> (32.6288, -2.8844) centre (32.1104, -5.2086) ccw
  line L37 (33.9073, -3.646) -> (60.7364, -34.498)
  line L38 (13.4831, -3.6754) -> (0, 11.7707)
  circle A106 centre (-11.8537, -67.2254) radius 1.7526 projected
  circle A107 centre (-11.8537, -67.2254) radius 4.7625 construction
  line L39 (-20.018, -66.9201) -> (-5.2592, -57.1461)
  line L40 (20.018, -66.9201) -> (5.2592, -57.1461)
  circle A108 centre (0, -53.975) radius 3.175
  circle A109 centre (0, -53.975) radius 1.7526 projected
  point P0 (18.4431, 0.2795)
  point P1 (13.4831, -3.6754)
  point P2 (-2.5228, -55.9027)
  point P3 (2.5228, -55.9027)
  point P4 (-8.5294, -69.3273)
  point P5 (8.5294, -69.3273)
  dimension "d179" = 146.05
  dimension "d181" = 19.05
  dimension "d180" = 15.875
  dimension "d182" = 3.175
  dimension "d185" = 360
  dimension "d187" = 6.35
  dimension "d188" = 6.35
  dimension "d189" = 9.525
  dimension "d190" = 45
  dimension "d191" = 6.35
  dimension "d192" = 0.7937
  dimension "d193" = 0.7937
  dimension "d194" = 0.7937
  dimension "d195" = 1.5875
  dimension "d196" = 9.525
  dimension "d201" = 6.35
  constraints: 40 end point, 25 point on circle, 19 centre point, 14 symmetric about line, 10 tangent, 6 coincident, 3 point on line, 2 vertical, 1 concentric, 1 vertical alignment, 27 other
  measures "d180" diameter of A87
  measures "d187" diameter of A94
  measures "d188" diameter of A95
  measures "d189" diameter of A97
  measures "d190" angle of L20 L21
  measures "d191" diameter of A98
  measures "d192" distance between parallel lines of L22 L24
  measures "d193" distance between parallel lines of L25 L23
  measures "d194" radial gap between concentric circles of A98 A99
  measures "d195" distance between parallel lines of L30 L26
  measures "d196" diameter of A107
  measures "d201" diameter of A108
extrude "Extrusion7" cut sketch "Sketch14" against normal blind 0.3969 contours L39 A89 L25 A99 L24 A94 L31 L38 A95 L36 A105 L37 L40 A88 A108 | A89 L21 A93 L23 A98 L22 A94 L24 A99 L25 | L37 A105 L36 A95 L34 A104 L35 A90 L33 A89
fillet "Fillet6" radius 1.5875 7 edges at (-20.018, 2.9766, 66.9201) (20.018, 2.9766, 66.9201) (0, 2.9766, -11.7707) (-61.4776, 2.9766, 33.1592) (61.4776, 2.9766, 33.1592) (-16.5662, 2.9766, -1.5114) (16.5662, 2.9766, -1.5114)
fillet "Fillet7" radius 3.175 2 edges at (2.5228, 2.9766, 55.9027) (-2.5228, 2.9766, 55.9027)
sketch "Sketch15" plane through (0, 0, 0) normal (0, -1, 0) x (1, 0, 0)
  point P0 (0, 65.0875)
  point P1 (-61.9019, 20.1131)
  point P2 (61.9019, 20.1131)
  point P3 (38.2575, -52.6569)
  point P4 (-38.2575, -52.6569)
hole "Hole8" at (0, 0, 65.0875) at (-61.9019, 0, 20.1131) at (61.9019, 0, 20.1131) at (38.2575, 0, -52.6569) at (-38.2575, 0, -52.6569) direction (0, 1, 0) diameter 3.7973 end through all
sketch "Sketch16" plane through (0, 3.175, 0) normal (0, 1, 0) x (1, 0, 0)
  circle A0 centre (20.7755, -50.424) radius 1.5875 projected
  circle A1 centre (19.4552, -56.6353) radius 1.5875 projected
  circle A2 centre (-20.7755, -50.424) radius 1.5875 projected
  circle A3 centre (-26.8147, -48.4618) radius 1.5875 projected
  circle A4 centre (-19.4552, -56.6353) radius 1.5875 projected
  circle A5 centre (-25.4944, -54.673) radius 3.175 projected
  circle A6 centre (31.5337, -52.7108) radius 1.5875 projected
  circle A7 centre (30.2134, -58.922) radius 1.5875 projected
  circle A8 centre (26.8147, -48.4618) radius 1.5875 projected
  circle A9 centre (-24.1742, -60.8843) radius 1.5875 projected
  circle A10 centre (-30.2134, -58.922) radius 1.5875 projected
  circle A11 centre (-31.5337, -52.7108) radius 1.5875 projected
  circle A12 centre (24.1742, -60.8843) radius 1.5875 projected
  circle A13 centre (25.4944, -54.673) radius 3.175 projected
  arc A14 (-4.7617, -56.8382) -> (-3.1745, -54.0317) centre (-6.349, -54.0884) ccw projected
  arc A15 (3.1745, -54.0317) -> (-3.1745, -54.0317) centre (0, -53.975) ccw projected
  arc A16 (3.1745, -54.0317) -> (4.7617, -56.8382) centre (6.349, -54.0884) ccw projected
  arc A17 (5.2592, -57.1461) -> (4.7617, -56.8382) centre (0, -65.0875) ccw projected
  line L0 (19.3941, -66.5069) -> (5.2592, -57.1461) projected
  arc A18 (19.3941, -66.5069) -> (20.742, -66.6993) centre (20.2706, -65.1834) ccw projected
  arc A19 (20.742, -66.6993) -> (60.8957, -34.216) centre (0, 0) ccw projected
  arc A20 (60.8957, -34.216) -> (60.6342, -32.3159) centre (59.5117, -33.4384) ccw projected
  line L1 (55.1667, -26.8483) -> (60.6342, -32.3159) projected
  arc A21 (54.7144, -26.3634) -> (55.1667, -26.8483) centre (61.9019, -20.1131) ccw projected
  line L2 (34.5063, -3.1251) -> (54.7144, -26.3634) projected
  arc A22 (34.5063, -3.1251) -> (32.8016, -2.1097) centre (32.1104, -5.2086) ccw projected
  line L3 (20.9486, 0.5339) -> (32.8016, -2.1097) projected
  arc A23 (20.9486, 0.5339) -> (19.027, -1.2062) centre (20.603, -1.0155) ccw projected
  arc A24 (13.4831, -3.6754) -> (19.027, -1.2062) centre (15.875, -1.5875) ccw projected
  line L4 (1.196, 10.4006) -> (13.4831, -3.6754) projected
  arc A25 (1.196, 10.4006) -> (-1.196, 10.4006) centre (0, 9.3567) ccw projected
  line L5 (-13.4831, -3.6754) -> (-1.196, 10.4006) projected
  arc A26 (-19.027, -1.2062) -> (-13.4831, -3.6754) centre (-15.875, -1.5875) ccw projected
  arc A27 (-19.027, -1.2062) -> (-20.9486, 0.5339) centre (-20.603, -1.0155) ccw projected
  line L6 (-32.8016, -2.1097) -> (-20.9486, 0.5339) projected
  arc A28 (-32.8016, -2.1097) -> (-34.5063, -3.1251) centre (-32.1104, -5.2086) ccw projected
  line L7 (-54.7144, -26.3634) -> (-34.5063, -3.1251) projected
  arc A29 (-55.1667, -26.8483) -> (-54.7144, -26.3634) centre (-61.9019, -20.1131) ccw projected
  line L8 (-60.6342, -32.3159) -> (-55.1667, -26.8483) projected
  arc A30 (-60.6342, -32.3159) -> (-60.8957, -34.216) centre (-59.5117, -33.4384) ccw projected
  arc A31 (-60.8957, -34.216) -> (-20.742, -66.6993) centre (0, 0) ccw projected
  arc A32 (-20.742, -66.6993) -> (-19.3941, -66.5069) centre (-20.2706, -65.1834) ccw projected
  line L9 (-5.2592, -57.1461) -> (-19.3941, -66.5069) projected
  arc A33 (-4.7617, -56.8382) -> (-5.2592, -57.1461) centre (0, -65.0875) ccw projected
  arc A34 (0.8193, 10.0718) -> (-0.8193, 10.0718) centre (0, 9.3567) ccw
  line L10 (0.8193, 10.0718) -> (13.1064, -4.0042)
  arc A35 (13.1064, -4.0042) -> (19.5234, -1.1461) centre (15.875, -1.5875) ccw
  arc A36 (20.8398, 0.0459) -> (19.5234, -1.1461) centre (20.603, -1.0155) ccw
  line L11 (20.8398, 0.0459) -> (32.6927, -2.5977)
  arc A37 (34.129, -3.4532) -> (32.6927, -2.5977) centre (32.1104, -5.2086) ccw
  line L12 (34.129, -3.4532) -> (54.3371, -26.6915)
  arc A38 (54.3371, -26.6915) -> (54.8131, -27.2019) centre (61.9019, -20.1131) ccw
  line L13 (54.8131, -27.2019) -> (60.2807, -32.6694)
  arc A39 (60.4598, -33.9711) -> (60.2807, -32.6694) centre (59.5117, -33.4384) ccw
  arc A40 (20.5936, -66.2218) -> (60.4598, -33.9711) centre (0, 0) ccw
  arc A41 (19.6702, -66.0901) -> (20.5936, -66.2218) centre (20.2706, -65.1834) ccw
  line L14 (19.6702, -66.0901) -> (5.5353, -56.7292)
  arc A42 (5.5353, -56.7292) -> (5.0117, -56.4051) centre (0, -65.0875) ccw
  arc A43 (3.6744, -54.0406) -> (5.0117, -56.4051) centre (6.349, -54.0884) ccw
  arc A44 (3.6744, -54.0406) -> (-3.6744, -54.0406) centre (0, -53.975) ccw construction
  arc A45 (-5.0117, -56.4051) -> (-3.6744, -54.0406) centre (-6.349, -54.0884) ccw
  arc A46 (-5.0117, -56.4051) -> (-5.5353, -56.7292) centre (0, -65.0875) ccw
  line L15 (-5.5353, -56.7292) -> (-19.6702, -66.0901)
  arc A47 (-20.5936, -66.2218) -> (-19.6702, -66.0901) centre (-20.2706, -65.1834) ccw
  arc A48 (-60.4598, -33.9711) -> (-20.5936, -66.2218) centre (0, 0) ccw
  arc A49 (-60.2807, -32.6694) -> (-60.4598, -33.9711) centre (-59.5117, -33.4384) ccw
  line L16 (-60.2807, -32.6694) -> (-54.8131, -27.2019)
  arc A50 (-54.8131, -27.2019) -> (-54.3371, -26.6915) centre (-61.9019, -20.1131) ccw
  line L17 (-54.3371, -26.6915) -> (-34.129, -3.4532)
  arc A51 (-32.6927, -2.5977) -> (-34.129, -3.4532) centre (-32.1104, -5.2086) ccw
  line L18 (-32.6927, -2.5977) -> (-20.8398, 0.0459)
  arc A52 (-19.5234, -1.1461) -> (-20.8398, 0.0459) centre (-20.603, -1.0155) ccw
  arc A53 (-19.5234, -1.1461) -> (-13.1064, -4.0042) centre (-15.875, -1.5875) ccw
  line L19 (-13.1064, -4.0042) -> (-0.8193, 10.0718)
  circle A54 centre (0, -53.975) radius 3.175
  arc A55 (1.3269, -56.8594) -> (-1.3269, -56.8594) centre (0, -65.0875) ccw
  line L20 (-2.9466, -52.7925) -> (-3.8664, -55.0847)
  arc A56 (3.1745, -54.0317) -> (-3.1745, -54.0317) centre (0, -53.975) ccw projected
  line L21 (0, -50.8) -> (0, -53.975) construction
  circle A57 centre (0, -53.975) radius 1.3891
  line L22 (2.9466, -52.7925) -> (3.8664, -55.0847)
  circle A58 centre (-15.875, -1.5875) radius 3.675
  circle A59 centre (-15.875, -1.5875) radius 3.175
  circle A60 centre (15.875, -1.5875) radius 3.675
  circle A61 centre (15.875, -1.5875) radius 3.175
  line L23 (-6.35, 1.4192) -> (6.35, 1.4192)
  line L24 (6.35, 1.4192) -> (6.35, 17.2942)
  line L25 (6.35, 17.2942) -> (-6.35, 17.2942)
  line L26 (-6.35, 17.2942) -> (-6.35, 1.4192)
  arc A62 (1.196, 10.4006) -> (-1.196, 10.4006) centre (0, 9.3567) ccw projected
  line L27 (-6.35, 1.4192) -> (6.35, 17.2942) construction
  line L28 (6.35, 1.4192) -> (-6.35, 17.2942) construction
  point P0 (3.1745, -54.0317)
  point P1 (-3.1745, -54.0317)
  point P2 (-6.35, 4.4962)
  point P3 (6.35, 4.4962)
  point P4 (13.4831, -3.6754)
  point P5 (19.027, -1.2062)
  point P6 (19.2632, -0.1641)
  point P7 (12.2661, -2.2812)
  point P8 (-12.2661, -2.2812)
  point P9 (-19.2632, -0.1641)
  point P10 (-19.027, -1.2062)
  dimension "d213" = 0.5
  dimension "d214" = 6.35
  dimension "d215" = 16.6687
  dimension "d216" = 2.7781
  dimension "d219" = 6.35
  dimension "d220" = 12.7
  dimension "d221" = 15.875
  constraints: 47 point on circle, 38 end point, 26 centre point, 6 coincident, 4 symmetric about line, 2 midpoint, 2 parallel, 2 tangent, 1 horizontal, 1 perpendicular, 1 vertical, 34 other
  measures "d213" distance between parallel lines of L5 L19
  measures "d214" diameter of A54
  measures "d215" diameter of A55
  measures "d216" diameter of A57
  measures "d219" diameter of A59
  measures "d220" distance of L25.end L24.end
  measures "d221" distance of L24.end L23.end
extrude "Extrusion8" add sketch "Sketch16" along normal blind 25.4 separate body contours A33 L9 A32 A31 A30 L8 A29 L7 A28 L6 A27 A58 A52 L18 A51 L17 A50 L16 A49 A48 A47 L15 A46 A45 L20 A15 A14 | A15 A54 A55 | L22 A43 A42 L14 A41 A40 A39 L13 A38 L12 A37 L11 A36 A60 A23 L3 A22 L2 A21 L1 A20 A19 A18 L0 A17 A16 A15 | A58 L5 A59 A27 | A27 A26 L5 A58 A53 | L5 L26 L19 A58 | L26 L25 L24 L4 A25 L5 | L5 A25 L4 L24 L10 A34 L19 L26 | A35 A60 L4 A24 A23 | A23 A61 L4 A60 | A60 L10 L24 L4
sketch "Sketch18" plane through (0, 3.175, 0) normal (0, 1, 0) x (1, 0, 0)
  circle A0 centre (0, 0) radius 76.2
  dimension "d228" = 152.4
  constraints: 1 centre point, 1 coincident
  measures "d228" diameter of A0
extrude "Extrusion10" cut sketch "Sketch18" against normal through all bodies 1
sketch "Sketch19" plane through (6.35, 28.575, -17.2942) normal (0, 0, -1) x (-1, 0, 0)
  line L0 (0, 0) -> (12.7, 0) projected
  line L1 (6.35, 0) -> (6.35, -25.4) construction
  line L2 (0, -25.4) -> (12.7, -25.4) projected
  line L3 (6.35, -6.35) -> (6.35, -19.05) construction
  line L4 (1.5875, -6.35) -> (1.5875, -19.05)
  line L5 (11.1125, -19.05) -> (11.1125, -6.35)
  arc A0 (11.1125, -6.35) -> (1.5875, -6.35) centre (6.35, -6.35) ccw
  arc A1 (1.5875, -19.05) -> (11.1125, -19.05) centre (6.35, -19.05) ccw
  point P0 (6.35, -12.7)
  dimension "d239" = 9.525
  dimension "d240" = 6.35
  constraints: 10 end point, 4 midpoint, 4 point on circle, 4 tangent, 2 centre point, 1 parallel, 1 point on line
  measures "d239" diameter of A1
  measures "d240" distance of point (6.35, -12.7) L3.start
extrude "Extrusion11" cut sketch "Sketch19" against normal blind 25.4 bodies 2
fillet "Fillet8" radius 0.7937 8 edges at (12.2661, 15.875, 2.2812) (19.2632, 15.875, 0.1641) (-12.2661, 15.875, 2.2812) (-19.2632, 15.875, 0.1641) (-3.1745, 15.875, 54.0317) (3.1745, 15.875, 54.0317) (1.3269, 15.875, 56.8594) (-1.3269, 15.875, 56.8594)
chamfer "Chamfer3" distance 1 angle 45 12 edges at (-3.6458, 25.2893, -6.8338) (0.0036, 26.9875, -10.4442) (3.6458, 25.2893, -6.8338) (4.7625, 15.875, -5.5545) (3.6458, 6.4607, -6.8338) (0.0036, 4.7625, -10.4442) (-3.6458, 6.4607, -6.8338) (-4.7625, 15.875, -5.5545) (0, 26.9875, -17.2942) (-4.7625, 15.875, -17.2942) (0, 4.7625, -17.2942) (4.7625, 15.875, -17.2942)
equation "\"d45\" = d42"
equation "\"d46\" = d41"
body "Solid1"
body "Solid2"
